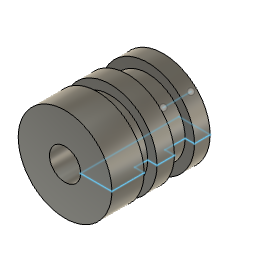
Sketch2 v1 (Autodesk Fusion 360 design; units mm, degrees)
Autodesk Fusion 360 part; units mm, degrees
sketch "Sketch1" plane through (0, 0, 0) normal (0, 0, 1) x (1, 0, 0)
  line L0 (18.2937, 44.1436) -> (28.2937, 44.1436)
  line L1 (28.2937, 44.1436) -> (28.2937, 39.1436)
  line L2 (28.2937, 39.1436) -> (25.2937, 39.1436)
  line L3 (25.2937, 39.1436) -> (25.2937, 32.6901)
  line L4 (25.2937, 32.6901) -> (28.2937, 32.6901)
  line L5 (28.2937, 32.6901) -> (28.2937, 27.1224)
  line L6 (28.2937, 27.1224) -> (25.2937, 27.1224)
  line L7 (25.2937, 27.1224) -> (25.2937, 22.9865)
  line L8 (25.2937, 22.9865) -> (28.2937, 22.9865)
  line L9 (28.2937, 22.9865) -> (28.2937, 12.6465)
  line L10 (18.2937, 44.1436) -> (18.2937, 12.6465)
  line L11 (28.2937, 12.6465) -> (18.2937, 12.6465)
  line L12 (13.2937, 44.1436) -> (13.2937, 53)
  dimension "d1" = 10
  dimension "d2" = 5
  dimension "d3" = 3
  dimension "d4" = 5
  constraint horizontal L0
  constraint perpendicular L0 L1
  constraint perpendicular L1 L2
  constraint perpendicular L0 L3
  constraint perpendicular L3 L4
  constraint perpendicular L4 L5
  constraint perpendicular L5 L6
  constraint perpendicular L6 L7
  constraint perpendicular L7 L8
  constraint perpendicular L8 L9
  constraint perpendicular L0 L10
  constraint perpendicular L10 L11
  measures "d1" distance of L0.start L0.end
  measures "d2" distance of L0.end L1.end
  measures "d3" distance of L1.end L2.end
  measures "d4" distance of L0.start L12.start
revolve "Revolve2" add sketch "Sketch1" angle 360 about axis through (13.2937, 53, 0) along (0, -1, 0)
